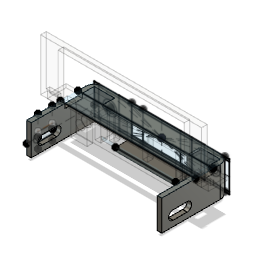
front_with_oled (Autodesk Fusion 360 design; units mm, degrees)
Autodesk Fusion 360 part; units mm, degrees
note: some values were not read from the file. Set by a fixed rule: which face or edge a step refers to.
sketch "Sketch1" plane through (0, 0, 0) normal (0, 0, 1) x (1, 0, 0) in component "front_bezel"
  line L0 (30, -6.75) -> (-30, -6.75)
  line L1 (-30, -6.75) -> (-30, 6.75)
  line L2 (-30, 6.75) -> (30, 6.75)
  line L3 (30, 6.75) -> (30, -6.75)
  line L4 (30, -6.75) -> (-30, 6.75) construction
  line L5 (-30, -6.75) -> (30, 6.75) construction
  line L6 (-28, 6.75) -> (-28, -6.75)
  line L7 (0, 6.75) -> (0, -6.75) construction
  line L8 (-30, 0) -> (30, 0) construction
  line L9 (28, 6.75) -> (28, -6.75)
  line L10 (23, 6.75) -> (23, -6.75) construction
  circle A0 centre (23, 0) radius 2
  circle A1 centre (23, 0) radius 3
  circle A2 centre (-23, 0) radius 3
  circle A3 centre (-23, 0) radius 2
  line L11 (-13.35, -5.8) -> (13.35, -5.8)
  line L12 (13.35, -5.8) -> (13.35, 5.8)
  line L13 (13.35, 5.8) -> (-13.35, 5.8)
  line L14 (-13.35, 5.8) -> (-13.35, -5.8)
  line L15 (-13.35, -5.8) -> (13.35, 5.8) construction
  line L16 (13.35, -5.8) -> (-13.35, 5.8) construction
  line L17 (13.35, 6.75) -> (13.35, -6.75)
  line L18 (-13.35, 6.75) -> (-13.35, -6.75)
  line L19 (-19, -6.75) -> (19, -6.75)
  line L20 (19, -6.75) -> (19, 6.75)
  line L21 (19, 6.75) -> (-19, 6.75)
  line L22 (-19, 6.75) -> (-19, -6.75)
  line L23 (-19, -6.75) -> (19, 6.75) construction
  line L24 (19, -6.75) -> (-19, 6.75) construction
  line L25 (30, -5.8) -> (-30, -5.8)
  line L26 (30, 5.8) -> (-30, 5.8)
  line L27 (13.35, -6.75) -> (-13.35, -6.75)
  line L28 (-13.35, -6.75) -> (-13.35, -8.25)
  line L29 (-13.35, -8.25) -> (13.35, -8.25)
  line L30 (13.35, -8.25) -> (13.35, -6.75)
  line L31 (8.35, 6.75) -> (8.35, -6.75)
  line L32 (-8.35, 6.75) -> (-8.35, -6.75)
  dimension "d1" = 60
  dimension "d2" = 13.5
  dimension "d3" = 2
  dimension "d13" = 5
  dimension "d14" = 4
  dimension "d15" = 6
  dimension "d23" = 26.7
  dimension "d24" = 11.6
  dimension "d59" = 38
  dimension "d122" = 1.5
  dimension "d210" = 5
  constraint horizontal L0
  constraint perpendicular L0 L1
  constraint parallel L0 L2
  constraint parallel L1 L3
  constraint coincident L4 origin
  constraint coincident L5 origin
  constraint coincident L2 L6.start
  constraint coincident L0 L6.end
  constraint perpendicular L0 L6
  constraint midpoint L2 L7.start
  constraint midpoint L0 L7.end
  constraint midpoint L1 L8.start
  constraint midpoint L3 L8.end
  constraint symmetric L6.start L7 L9.start
  constraint symmetric L6.end L7 L9.end
  constraint coincident L2 L10.start
  constraint coincident L0 L10.end
  constraint perpendicular L0 L10
  constraint midpoint L10 A0.centre
  constraint concentric A0 A1
  constraint symmetric L7 A0 A3
  constraint symmetric L7 A1 A2
  constraint horizontal L11
  constraint perpendicular L11 L12
  constraint parallel L11 L13
  constraint parallel L12 L14
  constraint coincident L15 origin
  constraint coincident L16 origin
  constraint coincident L2 L17.start
  constraint coincident L0 L17.end
  constraint perpendicular L0 L17
  constraint symmetric L7 L17.start L18.start
  constraint symmetric L7 L17.end L18.end
  constraint coincident L12.end L17
  constraint horizontal L19
  constraint perpendicular L19 L20
  constraint parallel L19 L21
  constraint parallel L20 L22
  constraint coincident L23 origin
  constraint coincident L24 origin
  constraint coincident L1.end L21
  constraint coincident L3 L25.start
  constraint coincident L1 L25.end
  constraint perpendicular L1 L25
  constraint coincident L11.start L25
  constraint coincident L3 L26.start
  constraint coincident L1 L26.end
  constraint perpendicular L1 L26
  constraint coincident L13.end L26
  constraint horizontal L27
  constraint vertical L28
  constraint horizontal L29
  constraint vertical L30
  constraint coincident L18.end L28
  constraint coincident L2 L31.start
  constraint coincident L27 L31.end
  constraint symmetric L7 L31.start L32.start
  constraint symmetric L7 L31.end L32.end
  measures "d1" distance of L1.end L2.end
  measures "d2" distance of L0.end L1.end
  measures "d3" distance of L1 L6
  measures "d13" distance of L9 L10
  measures "d14" diameter of A0
  measures "d15" diameter of A1
  measures "d23" distance of L12.end L13.end
  measures "d24" distance of L11.end L12.end
  measures "d59" distance of L20.end L21.end
  measures "d122" distance of L27 L29
  measures "d210" distance of L17 L31
extrude "Extrude1" add sketch "Sketch1" along normal blind 2 contours L0 L9 L20 L25 | L0 L17 L19 L20 L25 | L9 L20 L25 L26 | L0 L11 L17 L19 L25 L27 L31 | L12 L17 L20 L25 L26 | L2 L9 L20 L26 | L0 L11 L19 L25 L27 L31 L32 | L11 L12 L13 L17 L25 L26 L31 | L2 L17 L20 L21 L26 | L0 L11 L18 L19 L25 L27 L32 | L11 L13 L25 L26 L31 L32 | L2 L13 L17 L21 L26 L31 | L0 L18 L19 L22 L25 | L11 L13 L14 L18 L25 L26 L32 | L2 L13 L21 L26 L31 L32 | L0 L6 L22 L25 | L14 L18 L22 L25 L26 | L2 L13 L18 L21 L26 L32 | L6 L22 L25 L26 | L2 L18 L21 L22 L26 | L2 L6 L22 L26 | A0 | A1 | A2 | A3 makes body 1 in component "front_bezel"
extrude "Extrude2" add sketch "Sketch1" along normal blind 30 contours L0 L3 L9 L25 | L3 L9 L25 L26 | L2 L3 L9 L26 | L0 L1 L6 L25 | L1 L6 L25 L26 | L1 L2 L6 L26 bodies 1 in component "front_bezel"
sketch "Sketch2" plane through (-30, 0, 0) normal (-1, 0, 0) x (0, 0, 1) in component "front_bezel"
  line L0 (0, 6.75) -> (0, -6.75)
  line L1 (0, -6.75) -> (30, -6.75)
  line L2 (30, -6.75) -> (30, 6.75)
  line L3 (30, 6.75) -> (0, 6.75)
  line L4 (18.7, 6.75) -> (18.7, -6.75) construction
  line L5 (30, -2.25) -> (0, -2.25) construction
  line L6 (25, 6.75) -> (25, -6.75) construction
  line L7 (18.7, 0) -> (25, 0) construction
  line L8 (18.7, -4.25) -> (25, -4.25)
  arc A0 (25, -4.25) -> (25, -0.25) centre (25, -2.25) ccw
  line L9 (25, -0.25) -> (18.7, -0.25)
  arc A1 (18.7, -0.25) -> (18.7, -4.25) centre (18.7, -2.25) ccw
  line L10 (18.7, -2.25) -> (25, -2.25) construction
  dimension "d8" = 4.5
  dimension "d9" = 11.3
  dimension "d142" = 5
  dimension "d155" = 4
  constraint coincident L3 L4.start
  constraint coincident L1 L4.end
  constraint perpendicular L1 L4
  constraint coincident L2 L5.start
  constraint coincident L0 L5.end
  constraint perpendicular L0 L5
  constraint coincident L3 L6.start
  constraint coincident L1 L6.end
  constraint perpendicular L1 L6
  constraint perpendicular L6 L7
  constraint tangent L8 A0
  constraint tangent A0 L9
  constraint parallel L8 L9
  constraint tangent L9 A1
  constraint tangent L8 A1
  constraint coincident L5 A0.centre
  constraint coincident L6 A0.centre
  constraint perpendicular L6 L10
  constraint coincident L4 A1.centre
  measures "d8" distance of L1 L5
  measures "d9" distance of L2 L4
  measures "d142" distance of L2 L6
  measures "d155" diameter of A0
extrude "Extrude4" add sketch "Sketch1" along normal blind 3 contours A0 | A3 bodies 1 in component "front_bezel"
sketch "Sketch1 (2)" plane through (0, 0, 0) normal (0, 0, 1) x (1, 0, 0) in component "bezel_inner_holder"
  line L0 (27, -5.75) -> (-27, -5.75)
  line L1 (-27, -5.75) -> (-27, 5.75)
  line L2 (-27, 5.75) -> (27, 5.75)
  line L3 (27, 5.75) -> (27, -5.75)
  line L4 (27, -5.75) -> (-27, 5.75) construction
  line L5 (-27, -5.75) -> (27, 5.75) construction
  line L6 (-30, 6.75) -> (30, 6.75)
  line L7 (28, 6.75) -> (28, -6.75)
  circle A0 centre (-23, 0) radius 3.3
  line L8 (0, 5.75) -> (0, -5.75) construction
  line L9 (-27, 0) -> (27, 0) construction
  circle A1 centre (23, 0) radius 3.3
  line L10 (19.25, -5.25) -> (-19.25, -5.25)
  line L11 (-19.25, -5.25) -> (-19.25, 5.25)
  line L12 (-19.25, 5.25) -> (19.25, 5.25)
  line L13 (19.25, 5.25) -> (19.25, -5.25)
  line L14 (19.25, -5.25) -> (-19.25, 5.25) construction
  line L15 (-19.25, -5.25) -> (19.25, 5.25) construction
  line L16 (-16.75, 5.25) -> (-16.75, -5.25)
  line L17 (16.75, 5.25) -> (16.75, -5.25)
  line L18 (-19.25, 5.25) -> (-19.25, -5.25)
  line L19 (-19.25, 5.25) -> (-19.25, -5.75)
  line L20 (-19.25, -5.75) -> (-19.25, 5.25)
  line L21 (-19.25, 5.75) -> (-19.25, -5.75)
  line L22 (19.25, 5.75) -> (19.25, -5.75)
  line L23 (19.25, 6.75) -> (19.25, -5.75)
  line L24 (-19.25, -5.25) -> (-19.25, 6.75)
  line L25 (19.25, -5.25) -> (19.25, 6.75)
  line L26 (28, -6.75) -> (-30, -6.75)
  line L27 (-30, 6.75) -> (-30, -6.75)
  line L28 (19.25, 6.75) -> (19.25, -6.75)
  line L29 (-19.25, 6.75) -> (-19.25, -6.75)
  line L30 (1, 5.75) -> (1, -5.75)
  line L31 (-1, 5.75) -> (-1, -5.75)
  line L32 (15.75, 5.25) -> (15.75, -5.25)
  line L33 (13.75, 5.25) -> (13.75, -5.25)
  line L34 (-13.75, 5.25) -> (-13.75, -5.25)
  line L35 (-15.75, 5.25) -> (-15.75, -5.25)
  circle A2 centre (-23, 0) radius 2.25
  circle A3 centre (23, 0) radius 2.25
  circle A4 centre (-23, 0) radius 1.9
  circle A5 centre (23, 0) radius 1.9
  line L36 (8.75, 5.25) -> (8.75, -6.75)
  line L37 (-8.75, 5.25) -> (-8.75, -6.75)
  dimension "d18" = 1
  dimension "d19" = 1
  dimension "d20" = 6.6
  dimension "d32" = 38.5
  dimension "d33" = 0.5
  dimension "d34" = 2.5
  dimension "d35" = 4
  dimension "d55" = 1
  dimension "d95" = 1
  dimension "d96" = 2
  dimension "d117" = 4.5
  dimension "d204" = 3.8
  dimension "d212" = 5
  constraint horizontal L0
  constraint perpendicular L0 L1
  constraint parallel L0 L2
  constraint parallel L1 L3
  constraint coincident L4 origin
  constraint coincident L5 origin
  constraint midpoint L2 L8.start
  constraint midpoint L0 L8.end
  constraint midpoint L1 L9.start
  constraint midpoint L3 L9.end
  constraint symmetric A0 L8 A1
  constraint horizontal L10
  constraint perpendicular L10 L11
  constraint parallel L10 L12
  constraint parallel L11 L13
  constraint coincident L14 origin
  constraint coincident L15 origin
  constraint coincident L12 L16.start
  constraint coincident L10 L16.end
  constraint perpendicular L10 L16
  constraint coincident A0.centre L9
  constraint symmetric L8 L16.start L17.start
  constraint symmetric L8 L16.end L17.end
  constraint coincident L0 L19.end
  constraint coincident L11 L19.end
  constraint coincident L2 L21.start
  constraint perpendicular L0 L21
  constraint coincident L2 L22.start
  constraint coincident L0 L22.end
  constraint perpendicular L0 L22
  constraint coincident L10.start L22
  constraint coincident L6 L23.start
  constraint coincident L6 L24.end
  constraint perpendicular L6 L24
  constraint coincident L10.start L23
  constraint coincident L7.end L26.start
  constraint perpendicular L7 L26
  constraint coincident L6.start L27.start
  constraint perpendicular L6 L27
  constraint coincident L26 L28.end
  constraint perpendicular L26 L28
  constraint coincident L26 L29.end
  constraint perpendicular L26 L29
  constraint coincident L2 L30.start
  constraint coincident L0 L30.end
  constraint perpendicular L0 L30
  constraint symmetric L8 L30.start L31.start
  constraint symmetric L8 L30.end L31.end
  constraint coincident L12 L32.start
  constraint coincident L10 L32.end
  constraint perpendicular L0 L32
  constraint coincident L12 L33.start
  constraint coincident L10 L33.end
  constraint perpendicular L10 L33
  constraint symmetric L8 L32.start L35.start
  constraint symmetric L8 L32.end L35.end
  constraint symmetric L8 L33.start L34.start
  constraint symmetric L8 L33.end L34.end
  constraint concentric A0 A2
  constraint symmetric L8 A2 A3
  constraint concentric A0 A4
  constraint symmetric L8 A4 A5
  constraint coincident L12 L36.start
  constraint coincident L26 L36.end
  constraint perpendicular L26 L36
  constraint symmetric L8 L36.start L37.start
  constraint symmetric L8 L36.end L37.end
  measures "d18" distance of L2 L6
  measures "d19" distance of L3 L7
  measures "d20" diameter of A0
  measures "d32" distance of L11.end L12.end
  measures "d33" distance of L2 L12
  measures "d34" distance of L11 L16
  measures "d35" distance of L1 A0.centre
  measures "d55" distance of L8 L30
  measures "d95" distance of L17 L32
  measures "d96" distance of L32 L33
  measures "d117" diameter of A2
  measures "d204" diameter of A4
  measures "d212" distance of L33 L36
extrude "Extrude1'" add 1 faces at (-7.3333, -5.0774, 2) along direction (0, 0, 1) blind 8.4 separate body on bodies 1 makes body 2 in component "bezel_inner_holder"
extrude "Extrude1''" cut sketch "Sketch1" along normal up to surface (2 mm away) contours L11 L12 L13 L17 L25 L26 L31 | L11 L13 L25 L26 L31 L32 | L11 L13 L14 L18 L25 L26 L32 bodies 1 in component "front_bezel"
fillet "Fillet1" radius 4 2 edges at (-30, 0, 0) (30, 0, 0) on bodies 1 in component "front_bezel"
extrude "Extrude2'" add sketch "Sketch1" along normal blind 2.7 from surface at 2 contours L0 L11 L17 L19 L25 L27 L31 | L0 L11 L19 L25 L27 L31 L32 | L0 L11 L18 L19 L25 L27 L32 | L2 L13 L17 L21 L26 L31 | L2 L13 L21 L26 L31 L32 | L2 L13 L18 L21 L26 L32 bodies 1 in component "front_bezel"
extrude "Extrude2''" cut sketch "Sketch1 (2)" along normal blind 3 contours L10 L12 L33 L36 | L10 L12 L30 L36 | L10 L12 L17 L32 | L10 L12 L30 L31 | L10 L12 L32 L33 | L10 L12 L31 L37 | L10 L12 L34 L37 | L10 L12 L34 L35 | L10 L12 L16 L35 bodies 2 in component "bezel_inner_holder"
extrude "Extrude3" cut sketch "Sketch1 (2)" along normal up to surface (10.4 mm away) contours L10 L12 L13 L17 L22 L23 L25 L28 | L10 L11 L12 L16 L18 L19 L20 L21 L24 L29 bodies 2 in component "bezel_inner_holder"
sketch "Sketch2 (2)" plane through (0, 6.75, 0) normal (0, 1, 0) x (-1, 0, 0) in component "bezel_inner_holder"
  line L0 (-28, 2) -> (28, 2)
  line L1 (28, 2) -> (28, 10.4)
  line L2 (28, 10.4) -> (-28, 10.4)
  line L3 (-28, 10.4) -> (-28, 2)
  line L4 (-13.35, 4.7) -> (13.35, 4.7)
  line L5 (13.35, 2) -> (13.35, 4.7)
  line L6 (-13.35, 2) -> (-13.35, 4.7)
  line L7 (13.85, 2) -> (-13.85, 2)
  line L8 (-13.85, 2) -> (-13.85, 5.2)
  line L9 (-13.85, 5.2) -> (13.85, 5.2)
  line L10 (13.85, 5.2) -> (13.85, 2)
  line L11 (-19.25, 0) -> (-19.25, 10.4)
  line L12 (19.25, 0) -> (19.25, 10.4)
  line L13 (16.75, 0) -> (16.75, 10.4)
  line L14 (-16.75, 0) -> (-16.75, 10.4)
  line L15 (28, 5.2) -> (-28, 5.2)
  point P0 (-19.25, 0)
  point P1 (-16.75, 0)
  point P2 (16.75, 0)
  point P3 (19.25, 0)
  dimension "d40" = 0.5
  dimension "d41" = 0.5
  dimension "d42" = 0.5
  constraint horizontal L7
  constraint vertical L8
  constraint horizontal L9
  constraint vertical L10
  constraint coincident L0 L7.start
  constraint coincident P0 L11.start
  constraint coincident L2 L11.end
  constraint perpendicular L2 L11
  constraint coincident P3 L12.start
  constraint coincident L2 L12.end
  constraint perpendicular L2 L12
  constraint coincident P2 L13.start
  constraint coincident L2 L13.end
  constraint perpendicular L2 L13
  constraint coincident P1 L14.start
  constraint coincident L2 L14.end
  constraint perpendicular L2 L14
  constraint coincident L1 L15.start
  constraint coincident L3 L15.end
  constraint perpendicular L3 L15
  constraint coincident L9.end L15
  measures "d40" distance of L5 L10
  measures "d41" distance of L6 L8
  measures "d42" distance of L4 L9
extrude "Extrude4'" cut sketch "Sketch2 (2)" against normal blind 2 contours L0 L4 L5 L6 L7 L8 L9 L10 L15 | L0 L4 L5 L6 L7 bodies 2 in component "bezel_inner_holder"
extrude "Extrude5" cut sketch "Sketch2 (2)" along normal blind 2 from surface at -13.5 contours L0 L4 L5 L6 L7 L8 L9 L10 L15 | L0 L4 L5 L6 L7 bodies 2 in component "bezel_inner_holder"
extrude "Extrude6" cut sketch "Sketch1 (2)" along normal up to surface (5.2 mm away) contours L0 L26 L28 L36 | L0 L10 L22 L23 L28 L36 | L0 L26 L36 L37 | L0 L10 L30 L36 | L2 L12 L22 L23 L25 L28 L30 | L2 L6 L23 L24 L25 L28 L29 | L0 L10 L30 L31 | L2 L12 L30 L31 | L0 L10 L31 L37 | L0 L26 L29 L37 | L2 L12 L21 L24 L29 L31 | L0 L10 L19 L20 L21 L29 L37 bodies 2 in component "bezel_inner_holder"
extrude "Extrude7" cut 1 faces at (-4.6167, -1.5833, 3) along direction (0, 0, 1) up to surface (2.2 mm away) on bodies 2 bodies 2 in component "bezel_inner_holder"
extrude "Extrude8" cut 1 faces at (5.5833, -1.75, 5.2) along direction (0, 0, 1) blind 2.3 on bodies 2 bodies 2 in component "bezel_inner_holder"
extrude "Extrude9" add sketch "Sketch1 (2)" against normal blind 2.7 from surface at 7.5 contours L10 L12 L30 L31 bodies 2 in component "bezel_inner_holder"
extrude "Extrude3'" add sketch "Sketch1" along normal up to surface (7.2 mm away) contours L2 L17 L20 L21 L26 | L2 L18 L21 L22 L26 bodies 1 in component "front_bezel"
extrude "Extrude4''" add sketch "Sketch1" along normal up to surface (7.2 mm away) contours L2 L13 L17 L21 L26 L31 | L2 L13 L21 L26 L31 L32 | L2 L13 L18 L21 L26 L32 bodies 1 in component "front_bezel"
extrude "Extrude5'" add sketch "Sketch1" along normal up to surface (7.2 mm away) contours L0 L17 L19 L20 L25 | L0 L18 L19 L22 L25 bodies 1 in component "front_bezel"
extrude "Extrude6'" add 1 faces at (4.45, -6.4333, 4.7) along direction (0, 0, 1) up to surface (2.5 mm away) on bodies 1 bodies 1 in component "front_bezel"
sketch "Sketch1 (3)" plane through (0, 6.75, 0) normal (0, 1, 0) x (-1, 0, 0) in component "front_plate"
  line L0 (19.25, 7.5) -> (19.25, 2)
  line L1 (19.25, 2) -> (28, 2)
  line L2 (28, 2) -> (28, 10.4)
  line L3 (28, 10.4) -> (-28, 10.4)
  line L4 (-28, 10.4) -> (-28, 2)
  line L5 (-28, 2) -> (-19.25, 2)
  line L6 (-19.25, 2) -> (-19.25, 7.5)
  line L7 (-19.25, 7.5) -> (19.25, 7.5)
  line L8 (-28, 10.4) -> (28, 10.4)
  line L9 (28, 2) -> (28, 30)
  line L10 (-28, 2) -> (-28, 30)
  line L11 (-35.75, 14.05) -> (35.75, 14.05)
  line L12 (35.75, 14.05) -> (35.75, 6.75)
  line L13 (35.75, 6.75) -> (-35.75, 6.75)
  line L14 (-35.75, 6.75) -> (-35.75, 14.05)
  line L15 (-35.75, 14.05) -> (35.75, 6.75) construction
  line L16 (35.75, 14.05) -> (-35.75, 6.75) construction
  line L17 (27.7, 10.7) -> (-27.7, 10.7)
  line L18 (-27.7, 10.7) -> (-27.7, 13.2281)
  line L19 (-27.7, 13.2281) -> (27.7, 13.2281)
  line L20 (27.7, 13.2281) -> (27.7, 10.7)
  line L21 (27.25, 6.75) -> (27.25, 14.05)
  line L22 (27.25, 11.0945) -> (35.75, 11.0945)
  line L23 (0, 10.7) -> (0, 0) construction
  line L24 (-27.25, 11.0945) -> (-35.75, 11.0945)
  line L25 (-27.25, 6.75) -> (-27.25, 14.05)
  line L26 (35.75, 14.05) -> (27.7, 14.05)
  line L27 (27.7, 14.05) -> (27.7, 15.05)
  line L28 (27.7, 15.05) -> (35.75, 15.05)
  line L29 (35.75, 15.05) -> (35.75, 14.05)
  line L30 (35.75, 13.05) -> (27.7, 13.05)
  line L31 (-27.7, 15.05) -> (-35.75, 15.05)
  line L32 (-35.75, 13.05) -> (-27.7, 13.05)
  line L33 (-35.75, 15.05) -> (-35.75, 14.05)
  line L34 (-27.7, 14.05) -> (-27.7, 15.05)
  line L35 (-30.75, 6.75) -> (-30.75, 15.05)
  line L36 (30.75, 6.75) -> (30.75, 15.05)
  point P0 (0, 10.4)
  dimension "d68" = 71.5
  dimension "d69" = 7.3
  dimension "d71" = 0.3
  dimension "d72" = 0.3
  dimension "d73" = 0.3
  dimension "d74" = 8.5
  dimension "d76" = 2.9555
  dimension "d146" = 1
  dimension "d147" = 2
  dimension "d177" = 5
  constraint horizontal L11
  constraint perpendicular L11 L12
  constraint parallel L11 L13
  constraint parallel L12 L14
  constraint coincident L15 P0
  constraint coincident L16 P0
  constraint midpoint L8 P0
  constraint horizontal L17
  constraint horizontal L19
  constraint vertical L20
  constraint coincident L15 L18.end
  constraint parallel L10 L18
  constraint coincident L13 L21.start
  constraint coincident L11 L21.end
  constraint perpendicular L11 L21
  constraint coincident L21 L22.start
  constraint coincident L12 L22.end
  constraint perpendicular L12 L22
  constraint midpoint L17 L23.start
  constraint coincident L23.end origin
  constraint symmetric L21.start L23 L25.start
  constraint symmetric L21.end L23 L25.end
  constraint symmetric L22.start L23 L24.start
  constraint symmetric L22.end L23 L24.end
  constraint horizontal L26
  constraint vertical L27
  constraint horizontal L28
  constraint vertical L29
  constraint coincident L19.end L27
  constraint coincident L29 L30.start
  constraint coincident L27 L30.end
  constraint perpendicular L9 L30
  constraint symmetric L11.end L23 L11.start
  constraint symmetric L23 L26.end L34.start
  constraint symmetric L23 L27.end L31.start
  constraint symmetric L23 L28.end L31.end
  constraint symmetric L23 L30.start L32.start
  constraint symmetric L23 L30.end L32.end
  constraint coincident L13 L35.start
  constraint coincident L31 L35.end
  constraint perpendicular L31 L35
  constraint symmetric L23 L35.start L36.start
  constraint symmetric L23 L35.end L36.end
  measures "d68" distance of L12.end L13.end
  measures "d69" distance of L11 L13
  measures "d71" distance of L9 L20
  measures "d72" distance of L8 L17
  measures "d73" distance of L10 L18
  measures "d74" distance of L12 L21
  measures "d76" distance of L11 L22
  measures "d146" distance of L26 L28
  measures "d147" distance of L28 L30
  measures "d177" distance of L14 L35
extrude "Extrude1'''" add sketch "Sketch1 (3)" along normal blind 1.6 separate body contours L0 L3 L6 L7 L8 L13 L21 L25 | L2 L3 L8 L9 L13 L21 | L2 L9 L13 L22 L36 | L3 L8 L9 L17 L20 L21 L22 | L3 L8 L17 L21 L25 | L3 L4 L8 L10 L13 L25 | L12 L13 L22 L36 | L3 L8 L10 L17 L18 L24 L25 | L17 L20 L21 L22 | L17 L19 L21 L25 | L4 L10 L13 L24 L35 | L9 L20 L22 L30 | L9 L22 L30 L36 | L12 L22 L30 L36 | L17 L18 L24 L25 | L19 L20 L21 L22 | L13 L14 L24 L35 | L9 L11 L19 L20 L21 L26 L30 | L9 L11 L26 L30 L36 | L11 L12 L26 L30 L36 | L10 L24 L32 L35 | L10 L18 L24 L32 | L18 L19 L24 L25 | L11 L19 L21 L25 | L14 L24 L32 L35 | L10 L11 L32 L35 | L10 L11 L18 L19 L25 L32 | L11 L14 L32 L35 makes body 3 in component "front_plate"
extrude "Extrude2'''" add sketch "Sketch1 (3)" against normal up to surface (13.5 mm away) contours L17 L19 L21 L25 bodies 3 in component "front_plate"
extrude "Extrude7'" add sketch "Sketch1 (3)" along normal up to surface (1.6 mm away) contours L0 L6 L7 L13 bodies 3 in component "front_plate"
sketch "Sketch2 (3)" plane through (0, 0, 13.2281) normal (0, 0, 1) x (1, 0, 0) in component "front_plate"
  line L0 (-27.25, -6.75) -> (27.25, -6.75)
  line L1 (27.25, -6.75) -> (27.25, 6.75)
  line L2 (27.25, 6.75) -> (-27.25, 6.75)
  line L3 (-27.25, 6.75) -> (-27.25, -6.75)
sketch "Sketch3" plane through (0, 0, 3) normal (0, 0, 1) x (1, 0, 0) in component "front_plate"
  circle A0 centre (-23, 0) radius 2
  circle A1 centre (23, 0) radius 2
  circle A2 centre (-23, 0) radius 2
  line L0 (16.75, -5.25) -> (16.75, 5.25)
  line L1 (16.75, 5.25) -> (19.25, 5.25)
  line L2 (19.25, 5.25) -> (19.25, -5.25)
  line L3 (19.25, -5.25) -> (16.75, -5.25)
  line L4 (-19.25, -5.25) -> (-19.25, 5.25)
  line L5 (-19.25, 5.25) -> (-16.75, 5.25)
  line L6 (-16.75, 5.25) -> (-16.75, -5.25)
  line L7 (-16.75, -5.25) -> (-19.25, -5.25)
  circle A3 centre (-23, 0) radius 2
  circle A4 centre (23, 0) radius 2
  line L8 (-28, 6.75) -> (-28, -6.75)
  line L9 (-28, -6.75) -> (28, -6.75)
  line L10 (28, -6.75) -> (28, 6.75)
  line L11 (28, 6.75) -> (-28, 6.75)
  line L12 (-26.95, 6.75) -> (-19.95, 6.75)
  line L13 (-19.95, 6.75) -> (-19.95, -6.75)
  line L14 (-19.95, -6.75) -> (-26.95, -6.75)
  line L15 (-26.95, -6.75) -> (-26.95, 6.75)
  line L16 (-27.25, 6.75) -> (-27.25, -6.75)
  line L17 (19.8623, 6.75) -> (26.95, 6.75)
  line L18 (26.95, 6.75) -> (26.95, -6.75)
  line L19 (26.95, -6.75) -> (19.8623, -6.75)
  line L20 (19.8623, -6.75) -> (19.8623, 6.75)
  line L21 (27.25, -6.75) -> (27.25, 6.75)
  circle A5 centre (-23, 0) radius 2.25
  circle A6 centre (23, 0) radius 2.25
  dimension "d92" = 0.3
  dimension "d93" = 7
  dimension "d94" = 0.3
  constraint horizontal L12
  constraint vertical L13
  constraint horizontal L14
  constraint vertical L15
  constraint coincident L9 L13.end
  constraint coincident L11 L12.start
  constraint horizontal L17
  constraint vertical L18
  constraint horizontal L19
  constraint vertical L20
  constraint coincident L9 L18.end
  constraint coincident L11 L17.start
  measures "d92" distance of L15 L16
  measures "d93" distance of L13 L15
  measures "d94" distance of L18 L21
extrude "Extrude10" add sketch "Sketch1 (2)" along normal up to surface (2.7 mm away) from surface at 4.8 contours L10 L12 L32 L33 | L10 L12 L34 L35 bodies 2 in component "bezel_inner_holder"
extrude "Extrude11" cut 1 faces at (28, -2.25, 4.8) along direction (-1, 0, 0) blind 0.3 on bodies 2 bodies 2 in component "bezel_inner_holder"
extrude "Extrude12" cut 1 faces at (-28, 2.25, 4.8) along direction (1, 0, 0) blind 0.3 on bodies 2 bodies 2 in component "bezel_inner_holder"
sketch "Sketch1 (1)" plane through (0, 6.75, 0) normal (0, 1, 0) x (-1, 0, 0) in component "front_bezel"
  line L0 (-26, 0) -> (26, 0)
  arc A0 (26, 0) -> (30, 4) centre (26, 4) ccw
  line L1 (30, 4) -> (30, 30)
  line L2 (30, 30) -> (28, 30)
  line L3 (28, 30) -> (28, 2)
  line L4 (28, 2) -> (19, 2)
  line L5 (19, 2) -> (19, 7.2)
  line L6 (19, 7.2) -> (-19, 7.2)
  line L7 (-19, 7.2) -> (-19, 2)
  line L8 (-19, 2) -> (-28, 2)
  line L9 (-28, 2) -> (-28, 30)
  line L10 (-28, 30) -> (-30, 30)
  line L11 (-30, 30) -> (-30, 4)
  arc A1 (-30, 4) -> (-26, 0) centre (-26, 4) ccw
  line L12 (30, 7.2) -> (-30, 7.2)
  line L13 (30, 15) -> (-30, 15)
  dimension "d104" = 7.8
  constraint coincident L1 L12.start
  constraint coincident L11 L12.end
  constraint perpendicular L11 L12
  constraint coincident L6.end L12
  constraint coincident L1 L13.start
  constraint coincident L11 L13.end
  constraint perpendicular L11 L13
  measures "d104" distance of L12 L13
extrude "Extrude7''" cut sketch "Sketch1 (1)" against normal blind 2 contours L9 L11 L12 L13 | L1 L3 L12 L13 bodies 1 in component "front_bezel"
extrude "Extrude13" cut sketch "Sketch2 (2)" 1 faces at (24.8833, 6.75, 6.6333) along normal up to surface contours L1 L2 L12 L15 end surface through (0, 4.75, 0) normal (0, 1, 0) offset 0 on bodies 2 bodies 2 in component "bezel_inner_holder"
extrude "Extrude14" cut 3 faces at (14.4167, 5.25, 6.6) (-0.3333, 5.25, 5.7) (-14.4167, 5.25, 6.6) along direction (0, 1, 0) up to surface end surface through (0, 4.75, 0) normal (0, 1, 0) offset 0 on bodies 2 bodies 2 in component "bezel_inner_holder"
extrude "Extrude8'" cut sketch "Sketch3" along normal up to surface (2.8281 mm away) from surface at 7.4 contours L0 L1 L2 L3 | L4 L5 L6 L7 | L9 L11 L13 L20 bodies 3 in component "front_plate"
extrude "Extrude16" cut sketch "Sketch1 (2)" along normal up to surface (10.4 mm away) contours A2 | A3 | A4 | A5 bodies 2 in component "bezel_inner_holder"
extrude "Extrude8''" add sketch "Sketch1" along normal up to surface (7.2 mm away) contours L0 L19 L27 L28 L29 L30 bodies 1 in component "front_bezel"
sketch "Sketch2 (1)" plane through (0, 0, 7.2) normal (0, 0, 1) x (1, 0, 0) in component "front_bezel"
  line L0 (19, -5.8) -> (-19, -5.8)
  line L1 (-19, -5.8) -> (-19, -6.75)
  line L2 (-19, -6.75) -> (-13.35, -6.75)
  line L3 (-13.35, -6.75) -> (-13.35, -8.25)
  line L4 (-13.35, -8.25) -> (13.35, -8.25)
  line L5 (13.35, -8.25) -> (13.35, -6.75)
  line L6 (13.35, -6.75) -> (19, -6.75)
  line L7 (19, -6.75) -> (19, -5.8)
  line L8 (-13.35, -6.75) -> (13.35, -6.75)
  constraint coincident L2.end L3.start
  constraint coincident L5.end L6.start
extrude "Extrude9'" cut sketch "Sketch2 (1)" against normal up to surface (5.2 mm away) contours L0 L1 L2 L6 L7 L8 bodies 1 in component "front_bezel"
move_body "Move1" bodies 3 to x (1, 0, 0) y (0, 1, 0) z (0, 0, 1) at (0, -2, 0) in component "front_plate"
extrude "Extrude10'" cut sketch "Sketch3" along normal up to surface (2.5281 mm away) from surface at 7.7 contours A0 A2 A3 | A1 A4 bodies 3 in component "front_plate"
extrude "Extrude11'" cut 2 faces at (24.7874, -8.75, 12.3854) (-22.3833, -8.75, 12.3854) along direction (0, -1, 0) up to surface end surface through (13.35, -6.75, 4.7) normal (0, -1, 0) offset 0 on bodies 3 bodies 3 in component "front_plate"
extrude "Extrude12'" add sketch "Sketch1 (3)" against normal up to surface (2 mm away) contours L9 L11 L26 L28 L36 | L11 L26 L28 L29 L36 | L10 L11 L31 L35 | L11 L31 L33 L35 bodies 3 in component "front_plate"
extrude "Extrude14'" cut sketch "Sketch2" against normal up to surface (60 mm away) contours L8 A0 L9 A1 bodies 1 in component "front_bezel"
extrude "Extrude15" add sketch "Sketch1 (3)" along normal blind 2 contours L9 L11 L26 L28 L36 | L11 L26 L28 L29 L36 | L11 L31 L33 L35 bodies 3 in component "front_plate"
sketch "Sketch6" plane through (0, 8.75, 0) normal (0, 1, 0) x (-1, 0, 0) in component "front_plate"
  line L0 (35.75, 14.05) -> (35.75, 15.05)
  line L1 (35.75, 15.05) -> (28, 15.05)
  line L2 (28, 15.05) -> (28, 14.05)
  line L3 (35.75, 14.05) -> (28, 14.05)
  line L4 (28, 14.05) -> (28, 18.05)
  line L5 (28, 18.05) -> (35.75, 18.05)
  line L6 (35.75, 18.05) -> (35.75, 14.05)
  line L7 (27.7, 15.05) -> (35.75, 15.05)
  line L8 (35.75, 16.05) -> (28, 16.05)
  line L9 (28, 14.05) -> (35.75, 14.05)
  dimension "d160" = 3
  dimension "d161" = 2
  constraint horizontal L3
  constraint vertical L4
  constraint horizontal L5
  constraint vertical L6
  constraint coincident L0.start L3.start
  constraint coincident L1.end L4
  constraint coincident L6 L8.start
  constraint coincident L4 L8.end
  constraint perpendicular L4 L8
  measures "d160" distance of L5 L7
  measures "d161" distance of L5 L8
extrude "Extrude16'" add sketch "Sketch6" along normal blind 22 separate body contours L4 L5 L6 L8 makes body 4 in component "front_plate"
sketch "Sketch7" plane through (0, 8.75, 0) normal (0, 1, 0) x (-1, 0, 0) in component "front_plate"
  line L0 (-35.75, 15.05) -> (-35.75, 14.05)
  line L1 (-30.75, 15.05) -> (-35.75, 15.05)
  line L2 (-28, 13.05) -> (-35.75, 13.05)
  line L3 (-35.75, 13.05) -> (-35.75, 18.05)
  line L4 (-35.75, 18.05) -> (-28, 18.05)
  line L5 (-28, 18.05) -> (-28, 13.05)
  line L6 (-27.7, 15.05) -> (-35.75, 15.05)
  line L7 (-28, 15.55) -> (-35.75, 15.55)
  line L8 (-35.75, 14.05) -> (-30.75, 14.05)
  line L9 (-30.75, 14.05) -> (-30.75, 15.05)
  dimension "d166" = 3
  dimension "d167" = 2.5
  constraint horizontal L2
  constraint vertical L3
  constraint horizontal L4
  constraint vertical L5
  constraint coincident L0.start L3
  constraint coincident L5 L7.start
  constraint coincident L3 L7.end
  constraint perpendicular L3 L7
  measures "d166" distance of L4 L6
  measures "d167" distance of L4 L7
extrude "Extrude17" add sketch "Sketch6" sketch "Sketch7" against normal blind 1 contours L1 L4 L6 L7 L8 of sketch 2 contours L1 L3 L5 L6 L7 bodies 3 4 in component "front_plate"
extrude "Extrude18" add sketch "Sketch7" along normal up to surface (22 mm away) contours L3 L4 L5 L7 bodies 3 in component "front_plate"
extrude "Extrude19" add sketch "Sketch6" sketch "Sketch7" along normal up to surface contours L4 L5 L6 L8 of sketch 2 contours L3 L4 L5 L7 end surface through (0, 7.75, 0) normal (0, -1, 0) offset 0 bodies 3 in component "front_plate"
sketch "Sketch8" plane through (28, 0, 0) normal (-1, 0, 0) x (0, 0, 1) in component "front_plate"
  line L0 (15.05, 6.75) -> (14.05, 6.75)
  line L1 (14.05, 6.75) -> (14.05, 6.35)
  line L2 (14.05, 6.35) -> (14.05, 4.75)
  line L3 (14.05, 4.75) -> (15.05, 4.75)
  line L4 (15.05, 4.75) -> (15.05, 6.75)
sketch "Sketch9" plane through (0, 6.75, 0) normal (0, 1, 0) x (-1, 0, 0) in component "front_plate"
  line L0 (-28, 10.4) -> (-28, 2)
  line L1 (-28, 2) -> (-28, 30)
  line L2 (-30, 30) -> (-30, 4)
  line L3 (28, 2) -> (28, 30)
  line L4 (30, 30) -> (30, 0)
extrude "Extrude21" cut sketch "Sketch1 (3)" against normal blind 5 contours L9 L20 L22 L30 | L9 L22 L30 L36 | L19 L20 L21 L22 | L9 L11 L19 L20 L21 L26 L30 | L9 L11 L26 L30 L36 | L9 L11 L26 L28 L36 bodies 3 in component "front_plate"
extrude "Extrude22" cut sketch "Sketch1 (3)" along normal blind 7 contours L9 L11 L26 L30 L36 | L9 L11 L26 L28 L36 bodies 3 in component "front_plate"
extrude "Extrude23" cut 1 faces at (-28.9167, 8.0833, 15.05) along direction (0, 0, 1) up to surface (1 mm away) on bodies 3 bodies 3 in component "front_plate"
extrude "Extrude24" cut sketch "Sketch1 (3)" against normal up to surface (2 mm away) contours L10 L24 L32 L35 | L10 L18 L24 L32 | L10 L11 L32 L35 | L10 L11 L18 L19 L25 L32 bodies 3 in component "front_plate"
extrude "Extrude25" cut sketch "Sketch1 (3)" against normal blind 4 contours L10 L11 L32 L35 | L10 L11 L31 L35 bodies 3 in component "front_plate"
extrude "Extrude26" cut sketch "Sketch1 (3)" along normal blind 11 contours L10 L11 L32 L35 | L10 L11 L31 L35 bodies 3 in component "front_plate"
extrude "Extrude28" add 1 faces at (27.25, 5.8167, 13.5021) along direction (1, 0, 0) up to surface (0.45 mm away) on bodies 3 bodies 3 in component "front_plate"
sketch "Sketch10" plane through (28, 0, 0) normal (-1, 0, 0) x (0, 0, 1) in component "front_plate"
  line L0 (15.55, 8.75) -> (15.05, 8.75)
  line L1 (15.05, 8.75) -> (15.05, 7.75)
  line L2 (15.05, 7.75) -> (18.05, 7.75)
  line L3 (18.05, 7.75) -> (18.05, 30.75)
  line L4 (18.05, 30.75) -> (15.55, 30.75)
  line L5 (15.55, 30.75) -> (15.55, 8.75)
  line L6 (15.55, 28.75) -> (18.05, 28.75)
  dimension "d199" = 2
  constraint coincident L5 L6.start
  constraint coincident L3 L6.end
  constraint perpendicular L3 L6
  measures "d199" distance of L4 L6
extrude "Extrude31" add sketch "Sketch10" along normal up to surface (56 mm away) contours L3 L4 L5 L6 bodies 3 in component "front_plate"
extrude "Extrude32" add 1 faces at (-33.1667, 22.75, 16.05) along direction (0, 0, -1) up to surface (0.5 mm away) on bodies 3 bodies 3 in component "front_plate"
extrude "Extrude18'" add sketch "Sketch1 (2)" along normal blind 4.4 from surface at 2 contours A2 | A3 bodies 2 in component "bezel_inner_holder"
component "front_bezel" placed x (1, 0, 0) y (0, 1, 0) z (0, 0, 1) at (0, 0, 0)
component "bezel_inner_holder" placed x (1, 0, 0) y (0, 1, 0) z (0, 0, 1) at (0, 0, 0)
component "front_plate" placed x (1, 0, 0) y (0, 1, 0) z (0, 0, 1) at (0, 0, 0)
